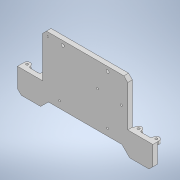
# Autodesk Inventor part: Motor Side Foot
Saved by Autodesk Inventor 2022 (Build 260153000, 153)
## iProperties
Created: 2022-05-29
Part Number: Motor Side Foot
Material: Generic
Document SubType Name: Modeling
Designer: Nick
Density: 1 g/cm^3
Appearance: Default
Author: Nick
Autodesk Inventor part; units mm, degrees
ref_plane "YZ Plane" through (0, 0, 0) normal (1, 0, 0) x (0, 1, 0)
ref_plane "XZ Plane" through (0, 0, 0) normal (0, 1, 0) x (-1, 0, 0)
ref_plane "XY Plane" through (0, 0, 0) normal (0, 0, 1) x (1, 0, 0)
sketch "Sketch1" plane through (0, 0, 0) normal (0, 0, 1) x (1, 0, 0)
  line L0 (-32.5, 0) -> (0, 0)
  line L1 (0, 0) -> (0, 58.05)
  line L2 (0, 58.05) -> (110, 58.05)
  line L3 (110, 58.05) -> (110, 0)
  line L4 (110, 0) -> (142.5, 0)
  line L5 (142.5, 0) -> (142.5, -30)
  line L6 (142.5, -30) -> (112.5, -30)
  line L7 (112.5, -30) -> (102.5, -20)
  line L8 (102.5, -20) -> (7.5, -20)
  line L9 (7.5, -20) -> (-2.5, -30)
  line L10 (-2.5, -30) -> (-32.5, -30)
  line L11 (-32.5, -30) -> (-32.5, 0)
  dimension "d0" = 135
  dimension "d1" = 135
  dimension "d2" = 110
  dimension "d3" = 58.05
  dimension "d4" = 30
  dimension "d5" = 32.5
  dimension "d6" = 20
  dimension "d7" = 30
  constraints: 24 end point, 4 collinear, 4 horizontal, 2 parallel, 2 perpendicular, 2 vertical, 1 coincident
  measures "d0" angle of L10 L9
  measures "d1" angle of L6 L7
  measures "d2" distance of L1.end L2.end
  measures "d3" distance of L0.end L1.end
  measures "d4" distance of L10.end L0.start
  measures "d5" distance of L0.start L0.end
  measures "d6" distance between parallel lines of L0 L8
  measures "d7" distance of L5.end L6.end
extrude "Extrusion1" add sketch "Sketch1" along normal blind 6
chamfer "Chamfer1" distance 5 angle 45 4 edges at (0, 58.05, 3) (110, 58.05, 3) (-32.5, -30, 3) (142.5, -30, 3)
sketch "Sketch2" plane through (110, 0, 0) normal (0, 1, 0) x (1, 0, 0)
  circle A0 centre (-138.5, 2.5) radius 1.5
  circle A1 centre (-115.5, 2.5) radius 1.5
  line L0 (-142.5, 0) -> (-142.5, -6) projected
  line L1 (-110, 0) -> (-142.5, 0) projected
  circle A2 centre (-138.5, 2.5) radius 4
  line L2 (-142.5, 0) -> (-112.5, 0) projected
  arc A3 (-142.5, 0) -> (-142.3846, 1.5461) centre (-144.8125, 0.95) ccw
  arc A4 (-134.5, 2.5) -> (-132, 0) centre (-132, 2.5) ccw
  arc A5 (-122, 0) -> (-119.5, 2.5) centre (-122, 2.5) ccw
  arc A6 (-111.5, 2.5) -> (-109, 0) centre (-109, 2.5) ccw
  circle A7 centre (-115.5, 2.5) radius 4
  line L3 (-109, 0) -> (-112.3775, 0)
  line L4 (-112.5, 0) -> (-102.5, 0) projected
  point P0 (-122, 0)
  point P1 (-132, 0)
  point P2 (-118.6225, 0)
  point P3 (-112.3775, 0)
  dimension "d13" = 3
  dimension "d14" = 3
  dimension "d15" = 4
  dimension "d16" = 27
  dimension "d17" = 2.5
  dimension "d18" = 8
  constraints: 13 point on circle, 8 centre point, 7 tangent, 4 equal radius, 4 point on line, 2 coincident, 2 end point, 2 horizontal alignment
  measures "d13" diameter of A1
  measures "d14" diameter of A0
  measures "d15" distance from line of L0 A0.centre
  measures "d16" distance from line of A1.centre L0
  measures "d17" distance from line of L1 A1.centre
  measures "d18" diameter of A2
extrude "Extrusion2" add sketch "Sketch2" against normal blind 4 contours L1 A7 A6 L3 | L1 A7 | L1 A5 A7 | L1 A2 A4 | L1 A2 | L1 A3 A2 picked at (-115.6011, 0.337) picked at (-138.4397, 0.337)
sketch "Sketch3" plane through (0, 0, 0) normal (0, 0, -1) x (-1, 0, 0)
  line L0 (-105, 58.05) -> (-5, 58.05) projected
  line L1 (0, 53.05) -> (0, 0) projected
  line L2 (-110, 0) -> (-110, 53.05) projected
  point P0 (-84, 52.55)
  point P1 (-26, 52.55)
  dimension "d21" = 5.5
  dimension "d22" = 26
  dimension "d23" = 26
  constraints: 1 horizontal alignment
  measures "d21" distance from line of L0 point (-26, 52.55)
  measures "d22" distance from line of L1 point (-26, 52.55)
  measures "d23" distance from line of L2 point (-84, 52.55)
hole "Hole1" at (84, 52.55, 0) at (26, 52.55, 0) direction (0, 0, 1) diameter 4 depth 24
sketch "Sketch4" plane through (7.5, -20, 0) normal (0, -1, 0) x (1, 0, 0)
  line L0 (84, 1.5) -> (82.5, 1.5)
  line L1 (82.5, 1.5) -> (82.5, 4.5)
  line L2 (82.5, 4.5) -> (84, 4.5)
  line L3 (84, 4.5) -> (84, 1.5)
  line L4 (87, 1.5) -> (87, 4.5)
  line L5 (-10, 0) -> (-10, 6) projected
  line L6 (95, 0) -> (95, 6) projected
  line L7 (63.5, 1.5) -> (62, 1.5)
  line L8 (62, 1.5) -> (62, 4.5)
  line L9 (62, 4.5) -> (63.5, 4.5)
  line L10 (63.5, 4.5) -> (63.5, 1.5)
  line L11 (66.5, 1.5) -> (66.5, 4.5)
  point P0 (-7.5, 0)
  point P1 (82.5, 3)
  point P2 (-10, 3)
  point P3 (87, 3)
  point P4 (84, 3)
  point P5 (63.5, 3)
  point P6 (66.5, 3)
  dimension "d31" = 1.5
  dimension "d32" = 3
  dimension "d33" = 3
  dimension "d35" = 8
  dimension "d36" = 1.5
  dimension "d37" = 3
  dimension "d38" = 3
  dimension "d39" = 16
  constraints: 20 end point, 6 horizontal alignment, 6 midpoint, 4 parallel, 2 horizontal, 2 perpendicular, 2 vertical
  measures "d31" distance of L1.end L2.end
  measures "d32" distance of L0.end L1.end
  measures "d33" distance between parallel lines of L4 L3
  measures "d35" distance between parallel lines of L6 L4
  measures "d36" distance of L7.start L7.end
  measures "d37" distance of L7.end L8.end
  measures "d38" distance between parallel lines of L10 L11
  measures "d39" distance between parallel lines of L1 L11
revolve "Revolution1" cut sketch "Sketch4" angle 360 about axis through (94.5, -20, 1.5) along (0, 0, 1) contours L0 L1 L2 L3
revolve "Revolution2" cut sketch "Sketch4" angle 360 about axis through (74, -20, 1.5) along (0, 0, 1) contours L7 L8 L9 L10
ref_plane "Work Plane1" through (55, 0, 6) normal (1, 0, 0) x (0, 0, -1)
mirror "Mirror1" about plane through (55, 0, 6) normal (1, 0, 0) of "Extrusion2"
sketch "Sketch5" plane through (0, 0, 6) normal (0, 0, 1) x (1, 0, 0)
  circle A0 centre (101.8237, 23.6209) radius 1.6
  circle A1 centre (70.8706, 26.6087) radius 1.6
  circle A2 centre (21.94, -11.4078) radius 1.6
  circle A3 centre (83.8562, -11.291) radius 1.6
  circle A4 centre (6.9179, 52.8175) radius 1.6
  circle A5 centre (70.8706, 26.6087) radius 4
  circle A6 centre (101.8237, 23.6209) radius 4
  circle A7 centre (83.8562, -11.291) radius 4
  circle A8 centre (21.94, -11.4078) radius 4
  circle A9 centre (6.9179, 52.8175) radius 4
  line L0 (109, 0) -> (109, -4) projected
  line L1 (7.5, -20) -> (102.5, -20) projected
  line L2 (110, 0) -> (102.5, -20)
  circle A10 centre (26, 52.55) radius 2 projected
  circle A11 centre (84, 52.55) radius 2 projected
  circle A12 centre (26, 52.55) radius 4
  circle A13 centre (84, 52.55) radius 4
  circle A14 centre (84, 52.55) radius 2 projected
  circle A15 centre (26, 52.55) radius 2 projected
  line L3 (105, 58.05) -> (110, 53.05) projected
  line L4 (105, 58.05) -> (5, 58.05) projected
  line L5 (0, 53.05) -> (5, 58.05) projected
  line L6 (0, 53.05) -> (0, 0) projected
  line L7 (0, 0) -> (-32.5, 0) projected
  line L8 (-32.5, 0) -> (-32.5, -25) projected
  line L9 (-27.5, -30) -> (-2.5, -30) projected
  line L10 (-2.5, -30) -> (7.5, -20) projected
  line L11 (7.5, -20) -> (102.5, -20) projected
  line L12 (102.5, -20) -> (112.5, -30) projected
  line L13 (112.5, -30) -> (137.5, -30) projected
  line L14 (142.5, -25) -> (142.5, 0) projected
  line L15 (142.5, 0) -> (110, 0) projected
  line L16 (110, 0) -> (110, 53.05) projected
  line L17 (0, 53.05) -> (5, 58.05) projected
  line L18 (105, 58.05) -> (5, 58.05) projected
  line L19 (105, 58.05) -> (110, 53.05) projected
  line L20 (142.5, -25) -> (137.5, -30) projected
  line L21 (-27.5, -30) -> (-32.5, -25) projected
  dimension "d41" = 8
  constraints: 12 centre point, 6 equal radius, 2 end point, 10 other
  measures "d41" diameter of A9
hole "Hole2" at (6.9179, 52.8175, 6) at (70.8706, 26.6087, 6) at (101.8237, 23.6209, 6) at (83.8562, -11.291, 6) at (21.94, -11.4078, 6) direction (0, 0, -1) diameter 2.5 depth 24
body "Solid1"
